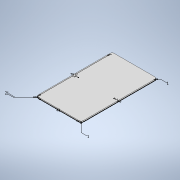
# Autodesk Inventor part: boden
Saved by Autodesk Inventor 2022 (Build 260153000, 153)
## iProperties
Created: 2022-04-04
Part Number: boden
Material: Generisch
Document SubType Name: Modeling
Designer: ga76xid
Density: 1 g/cm^3
Appearance: Vorgabe
Author: ga76xid
Autodesk Inventor part; units mm, degrees
ref_plane "YZ Plane" through (0, 0, 0) normal (1, 0, 0) x (0, 1, 0)
ref_plane "XZ Plane" through (0, 0, 0) normal (0, 1, 0) x (-1, 0, 0)
ref_plane "XY Plane" through (0, 0, 0) normal (0, 0, 1) x (1, 0, 0)
sketch "Skizze1" plane through (0, 0, 0) normal (0, 1, 0) x (-1, 0, 0)
  line L0 (1, 0) -> (40, 0)
  line L1 (41, 1) -> (41, 70)
  line L2 (40, 71) -> (1, 71)
  line L3 (0, 70) -> (0, 1)
  line L4 (42.2, 70.2) -> (42.2, 0.8)
  line L5 (40.2, -1.2) -> (0.8, -1.2)
  line L6 (-1.2, 0.8) -> (-1.2, 70.2)
  line L7 (0.8, 72.2) -> (40.2, 72.2)
  arc A0 (42.2, 70.2) -> (40.2, 72.2) centre (40.2, 70.2) ccw
  arc A1 (40.2, -1.2) -> (42.2, 0.8) centre (40.2, 0.8) ccw
  arc A2 (-1.2, 0.8) -> (0.8, -1.2) centre (0.8, 0.8) ccw
  arc A3 (0.8, 72.2) -> (-1.2, 70.2) centre (0.8, 70.2) ccw
  arc A4 (41, 70) -> (40, 71) centre (40, 70) ccw
  arc A5 (40, 0) -> (41, 1) centre (40, 1) ccw
  arc A6 (0, 1) -> (1, 0) centre (1, 1) ccw
  arc A7 (1, 71) -> (0, 70) centre (1, 70) ccw
  line L8 (1, 1) -> (1, 70)
  line L9 (1, 70) -> (40, 70)
  line L10 (40, 70) -> (40, 1)
  line L11 (40, 1) -> (1, 1)
  point P0 (0, 0)
  point P1 (41, 71)
  point P2 (41, 0)
  point P3 (0, 71)
  dimension "d0" = 41
  dimension "d1" = 71
  dimension "d2" = 1.2
  dimension "d3" = 2
  dimension "d4" = 1
  dimension "d5" = 1
  dimension "d6" = 1
  dimension "d9" = 1
  constraints: 24 end point, 16 point on circle, 16 tangent, 8 centre point, 8 point on line, 6 parallel, 4 equal radius, 3 perpendicular, 1 horizontal, 6 other
  measures "d0" distance of point (0, 71) point (41, 71)
  measures "d1" distance of point (41, 71) point (41, 0)
  measures "d2" distance between parallel lines of L1 L4
  measures "d3" radius of A0
  measures "d4" radius of A4
  measures "d5" radius of A6
  measures "d6" radius of A7
  measures "d9" distance between parallel lines of L3 L8
extrude "Extrusion1" add sketch "Skizze1" along normal blind 1 contours A6 L3 A7 L2 A4 L1 A5 L0 | L4 A1 L5 A2 L6 A3 L7 A0 | L8 L9 L10 L11
extrude "Extrusion2" add sketch "Skizze1" against normal blind 1 contours A6 L3 A7 L2 A4 L1 A5 L0
sketch "Skizze3" plane through (0, -1, 0) normal (0, -1, 0) x (1, 0, 0)
  arc A0 (-41, 1) -> (-40, 0) centre (-40, 1) ccw projected
  line L0 (-40, 0) -> (-1, 0) projected
  arc A1 (-1, 0) -> (0, 1) centre (-1, 1) ccw projected
  line L1 (0, 1) -> (0, 70) projected
  arc A2 (0, 70) -> (-1, 71) centre (-1, 70) ccw projected
  line L2 (-1, 71) -> (-40, 71) projected
  arc A3 (-40, 71) -> (-41, 70) centre (-40, 70) ccw projected
  line L3 (-41, 70) -> (-41, 1) projected
  line L4 (-1, 70) -> (-1, 1) projected
  line L5 (-1, 1) -> (-40, 1) projected
  line L6 (-40, 1) -> (-40, 70) projected
  line L7 (-40, 70) -> (-1, 70) projected
  line L8 (-1, 0.15) -> (-40, 0.15)
  arc A4 (-40.85, 1) -> (-40, 0.15) centre (-40, 1) ccw
  line L9 (-40.85, 1) -> (-40.85, 70)
  arc A5 (-40, 70.85) -> (-40.85, 70) centre (-40, 70) ccw
  line L10 (-40, 70.85) -> (-1, 70.85)
  arc A6 (-0.15, 70) -> (-1, 70.85) centre (-1, 70) ccw
  line L11 (-0.15, 70) -> (-0.15, 1)
  arc A7 (-1, 0.15) -> (-0.15, 1) centre (-1, 1) ccw
  point P0 (0, 0)
  dimension "d12" = 0.15
  constraints: 8 end point, 8 point on circle, 4 centre point, 7 other
  measures "d12" distance between parallel lines of L0 L8
extrude "Extrusion3" cut sketch "Skizze3" against normal blind 1 contours L3 A3 L2 A2 L1 A1 L0 A0
